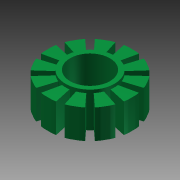
# Autodesk Inventor part: anchor
Saved by Autodesk Inventor 2012 (Build 160160000, 160)
## iProperties
Created: 2014-07-09
Part Number: anchor
Material: Default
Document SubType Name: Modeling
Designer: Anon
Density: 1 g/cm^3
Author: Anon
Autodesk Inventor part; units mm, degrees
ref_plane "YZ Plane" through (0, 0, 0) normal (1, 0, 0) x (0, 1, 0)
ref_plane "XY Plane" through (0, 0, 0) normal (0, 0, 1) x (1, 0, 0)
sketch "Sketch1" plane through (0, 0, 0) normal (0, 0, 1) x (1, 0, 0)
  circle A0 centre (0, 0) radius 8
  dimension "d0" = 16
  constraints: 1 centre point, 1 coincident
  measures "d0" diameter of A0
extrude "Extrusion1" add sketch "Sketch1" along normal blind 11.5
ref_plane "Work Plane1" through (0, -8, 0) normal (0, 1, 0) x (-1, 0, 0)
sketch "Sketch2" plane through (0, -8, 0) normal (0, 1, 0) x (-1, 0, 0)
  line L0 (-1.25, 1) -> (1.25, 1)
  line L1 (1.25, 1) -> (1.25, 10.5)
  line L2 (1.25, 10.5) -> (-1.25, 10.5)
  line L3 (-1.25, 10.5) -> (-1.25, 1)
  point P0 (0, 0)
  dimension "d3" = 2.5
  dimension "d4" = 9.5
  dimension "d5" = 10.5
  dimension "d6" = 1.25
  constraints: 8 end point, 2 parallel, 1 horizontal, 1 perpendicular
  measures "d3" distance of L2.end L1.end
  measures "d4" distance of L1.end L0.end
  measures "d5" distance from line of L2 point (0, 0)
  measures "d6" distance from line of L3 point (0, 0)
extrude "Extrusion2" add sketch "Sketch2" along normal blind 1
ref_plane "Work Plane2" through (0, -13.7, 0) normal (0, -1, 0) x (1, 0, 0)
sketch "Sketch4" plane through (0, -13.7, 0) normal (0, -1, 0) x (1, 0, 0)
  line L0 (-2.5, 10.5) -> (2.5, 10.5)
  line L1 (2.5, 10.5) -> (2.5, 1)
  line L2 (2.5, 1) -> (-2.5, 1)
  line L3 (-2.5, 1) -> (-2.5, 10.5)
  point P0 (0, 0)
  dimension "d10" = 9.5
  dimension "d11" = 1
  dimension "d12" = 5
  dimension "d13" = 2.5
  constraints: 8 end point, 2 parallel, 1 horizontal, 1 perpendicular
  measures "d10" distance between parallel lines of L2 L0
  measures "d11" distance from line of point (0, 0) L2
  measures "d12" distance between parallel lines of L1 L3
  measures "d13" distance from line of point (0, 0) L3
loft "Loft1" add profiles "Sketch4" section 2 edges at (-0.625, -8, 10.5) (-1.25, -8, 5.75) (-0.625, -8, 1) (0.625, -8, 1) (1.25, -8, 5.75) (0.625, -8, 10.5)
pattern_circular "Circular Pattern1" count 12 over 360 about axis through (0, 0, -10) along (0, 0, 1) of "Extrusion2", "Loft1"
sketch "Sketch5" plane through (0, 0, 11.5) normal (0, 0, 1) x (1, 0, 0)
  circle A0 centre (0, 0) radius 8 projected
  circle A1 centre (0, 0) radius 13.75
  circle A2 centre (0, 0) radius 17.044
  dimension "d21" = 27.5
  constraints: 2 centre point, 2 coincident
  measures "d21" diameter of A1
extrude "Extrusion3" cut sketch "Sketch5" along normal through all both and the other way through all contours A2
sketch "Sketch6" plane through (0, 0, 0) normal (0, 0, -1) x (-1, 0, 0)
  circle A0 centre (0, 0) radius 8 projected
  circle A1 centre (0, 0) radius 6.5
  dimension "d24" = 13
  constraints: 1 centre point, 1 coincident
  measures "d24" diameter of A1
extrude "Extrusion4" cut sketch "Sketch6" against normal through all contours A1
ref_plane "Work Plane3" through (6.85, -11.8645, 0) normal (0.5, -0.8660254, 0) x (0.8660254, 0.5, 0)
ref_plane "Work Plane4" through (11.8645, -6.85, 0) normal (0.8660254, -0.5, 0) x (0.5, 0.8660254, 0)
ref_plane "Work Plane5" through (13.7, 0, 0) normal (1, 0, 0) x (0, 1, 0)
ref_plane "Work Plane6" through (11.8645, 6.85, 0) normal (0.8660254, 0.5, 0) x (-0.5, 0.8660254, 0)
ref_plane "Work Plane7" through (6.85, 11.8645, 0) normal (0.5, 0.8660254, 0) x (-0.8660254, 0.5, 0)
ref_plane "Work Plane8" through (0, 13.7, 0) normal (0, 1, 0) x (-1, 0, 0)
ref_plane "Work Plane9" through (-6.85, 11.8645, 0) normal (-0.5, 0.8660254, 0) x (-0.8660254, -0.5, 0)
ref_plane "Work Plane10" through (-11.8645, 6.85, 0) normal (-0.8660254, 0.5, 0) x (-0.5, -0.8660254, 0)
ref_plane "Work Plane11" through (-13.7, 0, 0) normal (-1, 0, 0) x (0, -1, 0)
ref_plane "Work Plane12" through (-11.8645, -6.85, 0) normal (-0.8660254, -0.5, 0) x (0.5, -0.8660254, 0)
ref_plane "Work Plane13" through (-6.85, -11.8645, 0) normal (-0.5, -0.8660254, 0) x (0.8660254, -0.5, 0)
body "Solid1"
